Autodesk Fusion 360 part; units mm, degrees
(part 14 of 14)
sketch "Gear Tooth" plane through (0, 0, 0) normal (0, 0, 1) x (1, 0, 0)
  spline S0 degree 5 poles (44.1435, -1.3961) (44.1546, -1.396) (44.1768, -1.3957) (44.2102, -1.3951) (44.2546, -1.3938) (44.3102, -1.3914) (44.3658, -1.3882) (44.4214, -1.3842) (44.477, -1.3795) (44.5325, -1.3742) (44.5881, -1.3682) (44.6437, -1.3617) (44.6992, -1.3548) (44.7548, -1.3474) (44.8103, -1.3396) (44.8658, -1.3315) (44.9213, -1.3229) (44.9768, -1.314) (45.0323, -1.3047) (45.0878, -1.295) (45.1432, -1.285) (45.1987, -1.2746) (45.2541, -1.2639) (45.3095, -1.2528) (45.3649, -1.2415) (45.4203, -1.2298) (45.4756, -1.2179) (45.5309, -1.2056) (45.5863, -1.1931) (45.6416, -1.1803) (45.6969, -1.1672) (45.7521, -1.1538) (45.8074, -1.1401) (45.8626, -1.1262) (45.9178, -1.112) (45.973, -1.0975) (46.0282, -1.0828) (46.0833, -1.0678) (46.1384, -1.0526) (46.1935, -1.0371) (46.2486, -1.0214) (46.3037, -1.0055) (46.3587, -0.9893) (46.4137, -0.9728) (46.4687, -0.9562) (46.5237, -0.9393) (46.5786, -0.9222) (46.6336, -0.9048) (46.6885, -0.8872) (46.7433, -0.8694) (46.7982, -0.8514) (46.853, -0.8332) (46.9078, -0.8147) (46.9626, -0.796) (47.0173, -0.7771) (47.0721, -0.758) (47.1268, -0.7387) (47.1814, -0.7192) (47.2361, -0.6995) (47.2907, -0.6796) (47.3453, -0.6595) (47.3999, -0.6391) (47.4544, -0.6186) (47.5089, -0.5979) (47.5634, -0.5769) (47.6179, -0.5558) (47.6723, -0.5345) (47.7267, -0.513) (47.7811, -0.4913) (47.8354, -0.4694) (47.8898, -0.4473) (47.9332, -0.4295) (47.9658, -0.416) (47.9875, -0.407) (47.9983, -0.4025) knots 0 0 0 0 0 0 0.01428571 0.02857143 0.04285714 0.05714286 0.07142857 0.08571429 0.1 0.11428571 0.12857143 0.14285714 0.15714286 0.17142857 0.18571429 0.2 0.21428571 0.22857143 0.24285714 0.25714286 0.27142857 0.28571429 0.3 0.31428571 0.32857143 0.34285714 0.35714286 0.37142857 0.38571429 0.4 0.41428571 0.42857143 0.44285714 0.45714286 0.47142857 0.48571429 0.5 0.51428571 0.52857143 0.54285714 0.55714286 0.57142857 0.58571429 0.6 0.61428571 0.62857143 0.64285714 0.65714286 0.67142857 0.68571429 0.7 0.71428571 0.72857143 0.74285714 0.75714286 0.77142857 0.78571429 0.8 0.81428571 0.82857143 0.84285714 0.85714286 0.87142857 0.88571429 0.9 0.91428571 0.92857143 0.94285714 0.95714286 0.97142857 0.98571429 1 1 1 1 1 1
  spline S1 degree 5 poles (44.1435, 1.3961) (44.1546, 1.396) (44.1768, 1.3957) (44.2102, 1.3951) (44.2546, 1.3938) (44.3102, 1.3914) (44.3658, 1.3882) (44.4214, 1.3842) (44.477, 1.3795) (44.5325, 1.3742) (44.5881, 1.3682) (44.6437, 1.3617) (44.6992, 1.3548) (44.7548, 1.3474) (44.8103, 1.3396) (44.8658, 1.3315) (44.9213, 1.3229) (44.9768, 1.314) (45.0323, 1.3047) (45.0878, 1.295) (45.1432, 1.285) (45.1987, 1.2746) (45.2541, 1.2639) (45.3095, 1.2528) (45.3649, 1.2415) (45.4203, 1.2298) (45.4756, 1.2179) (45.5309, 1.2056) (45.5863, 1.1931) (45.6416, 1.1803) (45.6969, 1.1672) (45.7521, 1.1538) (45.8074, 1.1401) (45.8626, 1.1262) (45.9178, 1.112) (45.973, 1.0975) (46.0282, 1.0828) (46.0833, 1.0678) (46.1384, 1.0526) (46.1935, 1.0371) (46.2486, 1.0214) (46.3037, 1.0055) (46.3587, 0.9893) (46.4137, 0.9728) (46.4687, 0.9562) (46.5237, 0.9393) (46.5786, 0.9222) (46.6336, 0.9048) (46.6885, 0.8872) (46.7433, 0.8694) (46.7982, 0.8514) (46.853, 0.8332) (46.9078, 0.8147) (46.9626, 0.796) (47.0173, 0.7771) (47.0721, 0.758) (47.1268, 0.7387) (47.1814, 0.7192) (47.2361, 0.6995) (47.2907, 0.6796) (47.3453, 0.6595) (47.3999, 0.6391) (47.4544, 0.6186) (47.5089, 0.5979) (47.5634, 0.5769) (47.6179, 0.5558) (47.6723, 0.5345) (47.7267, 0.513) (47.7811, 0.4913) (47.8354, 0.4694) (47.8898, 0.4473) (47.9332, 0.4295) (47.9658, 0.416) (47.9875, 0.407) (47.9983, 0.4025) knots 0 0 0 0 0 0 0.01428571 0.02857143 0.04285714 0.05714286 0.07142857 0.08571429 0.1 0.11428571 0.12857143 0.14285714 0.15714286 0.17142857 0.18571429 0.2 0.21428571 0.22857143 0.24285714 0.25714286 0.27142857 0.28571429 0.3 0.31428571 0.32857143 0.34285714 0.35714286 0.37142857 0.38571429 0.4 0.41428571 0.42857143 0.44285714 0.45714286 0.47142857 0.48571429 0.5 0.51428571 0.52857143 0.54285714 0.55714286 0.57142857 0.58571429 0.6 0.61428571 0.62857143 0.64285714 0.65714286 0.67142857 0.68571429 0.7 0.71428571 0.72857143 0.74285714 0.75714286 0.77142857 0.78571429 0.8 0.81428571 0.82857143 0.84285714 0.85714286 0.87142857 0.88571429 0.9 0.91428571 0.92857143 0.94285714 0.95714286 0.97142857 0.98571429 1 1 1 1 1 1
  arc A0 (47.9983, -0.4025) -> (47.9983, 0.4025) centre (0, 0) ccw
  line L0 (44.1435, 1.3961) -> (44.1435, -1.3961)
  point P0 (44.4179, -1.3843)
  point P1 (44.6928, -1.3555)
  point P2 (44.968, -1.3153)
  point P3 (45.2434, -1.2659)
  point P4 (45.519, -1.2082)
  point P5 (45.7946, -1.1432)
  point P6 (46.0703, -1.0713)
  point P7 (46.346, -0.993)
  point P8 (46.6217, -0.9085)
  point P9 (46.8973, -0.8182)
  point P10 (47.1728, -0.7223)
  point P11 (47.4482, -0.6209)
  point P12 (47.7233, -0.5143)
  point P13 (44.4179, 1.3843)
  point P14 (44.6928, 1.3555)
  point P15 (44.968, 1.3153)
  point P16 (45.2434, 1.2659)
  point P17 (45.519, 1.2082)
  point P18 (45.7946, 1.1432)
  point P19 (46.0703, 1.0713)
  point P20 (46.346, 0.993)
  point P21 (46.6217, 0.9085)
  point P22 (46.8973, 0.8182)
  point P23 (47.1728, 0.7223)
  point P24 (47.4482, 0.6209)
  point P25 (47.7233, 0.5143)
extrude "Extrude2" add sketch "Gear Tooth" along normal blind 6
fillet "Fillet1" radius 0.38 2 edges at (45.829, 1.1346, 3) (45.829, -1.1346, 3)
pattern_circular "C-Pattern1" count 94 over 360 about axis through (0, 0, 0) along (0, 0, 1) of "Extrude2", "Fillet1"
sketch "Diametrial Pitch Circle" plane through (0, 0, 0) normal (0, 0, 1) x (1, 0, 0)
  circle A0 centre (0, 0) radius 47 construction
named bodies: "Spur Gear (94 teeth)"

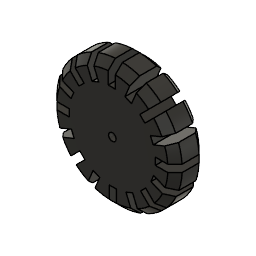
design "car project wheels"
part number: 2026-02-16-19-34-30-202
Autodesk Fusion 360 part; units mm, degrees
sketch "Sketch1" plane through (0, 0, 0) normal (0, 0, 1) x (1, 0, 0)
  circle A0 centre (0, 0) radius 2.1
  circle A1 centre (0, 0) radius 35
  dimension "d1" = 4.2
  dimension "d2" = 70
  constraint coincident A0.centre A1.centre
  measures "d1" diameter of A0
  measures "d2" diameter of A1
extrude "Extrude1" add sketch "Sketch1" along normal blind 17.5
chamfer "Chamfer1" distance 4 angle 45 2 edges at (-32.6315, -12.6565, 17.5) (-32.6315, -12.6565, 0)
sketch "Sketch2" plane through (0, 0, 0) normal (0, 0, 1) x (1, 0, 0)
sketch "Sketch3" plane through (0, 0, 0) normal (0, 0, 1) x (1, 0, 0)
sketch "Sketch5" plane through (0, 0, 0) normal (0, 0, 1) x (1, 0, 0)
  line L0 (-0.313, 36) -> (1.687, 36)
  line L1 (1.687, 36) -> (1.687, 24)
  line L2 (1.687, 24) -> (-2.313, 24)
  line L3 (-2.313, 24) -> (-2.313, 36)
  line L4 (-2.313, 36) -> (-0.313, 36)
  dimension "d17" = 2
  dimension "d18" = 12
  dimension "d19" = 4
  dimension "d20" = 12
  constraint horizontal L0
  constraint perpendicular L0 L1
  constraint perpendicular L1 L2
  constraint perpendicular L2 L3
  measures "d17" distance of L0.start L0.end
  measures "d18" distance of L0.end L1.end
  measures "d19" distance of L1.end L2.end
  measures "d20" distance of L2.end L3.end
extrude "Extrude3" cut sketch "Sketch5" along normal blind 45
pattern_circular "C-Pattern3" count 16 over 360 about axis through (0, 0, 0) along (0, 0, 1) of "Extrude3"
sketch "Sketch6" plane through (0, 0, 0) normal (0, 0, 1) x (1, 0, 0)

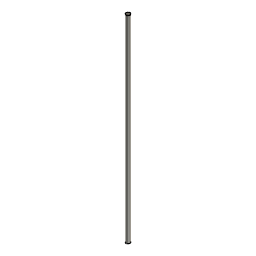
design "Axle"
part number: 2026-03-02-11-54-45-351
Autodesk Fusion 360 part; units mm, degrees
sketch "Sketch1" plane through (0, 0, 0) normal (0, 0, 1) x (1, 0, 0)
  circle A0 centre (0, 0) radius 2
  dimension "d1" = 4
  constraint coincident A0.centre origin
  measures "d1" diameter of A0
extrude "Extrude1" add sketch "Sketch1" along normal blind 190

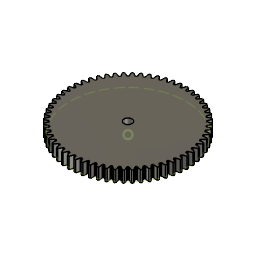
design "60 compound gear"
description: Spur Gear; Module: 1.0; Num Teeth: 60; Pressure Angle: 20.0; Backlash: 0.00 mm
part number: 2026-09-03-00-53-56-789
Autodesk Fusion 360 part; units mm, degrees
sketch "Base Circle" plane through (0, 0, 0) normal (0, 0, 1) x (1, 0, 0)
  circle A0 centre (0, 0) radius 28.843
  circle A1 centre (0, 0) radius 2.1
extrude "Extrude1" add sketch "Base Circle" along normal blind 6
sketch "Gear Tooth" plane through (0, 0, 0) normal (0, 0, 1) x (1, 0, 0)
  spline S0 degree 5 poles (28.167, -1.1579) (28.1751, -1.1579) (28.1914, -1.1578) (28.2159, -1.1575) (28.2485, -1.1567) (28.2892, -1.1551) (28.33, -1.1529) (28.3707, -1.1501) (28.4115, -1.1467) (28.4523, -1.1427) (28.493, -1.1383) (28.5338, -1.1335) (28.5746, -1.1284) (28.6154, -1.1228) (28.6561, -1.117) (28.6969, -1.1109) (28.7376, -1.1045) (28.7783, -1.0977) (28.8191, -1.0907) (28.8598, -1.0834) (28.9005, -1.0758) (28.9412, -1.0679) (28.9819, -1.0597) (29.0226, -1.0513) (29.0633, -1.0427) (29.104, -1.0338) (29.1446, -1.0247) (29.1853, -1.0153) (29.2259, -1.0057) (29.2665, -0.9959) (29.3071, -0.9858) (29.3477, -0.9755) (29.3883, -0.965) (29.4289, -0.9543) (29.4694, -0.9434) (29.5099, -0.9323) (29.5505, -0.921) (29.591, -0.9094) (29.6315, -0.8977) (29.672, -0.8858) (29.7124, -0.8737) (29.7529, -0.8614) (29.7933, -0.8488) (29.8337, -0.8361) (29.8741, -0.8233) (29.9145, -0.8102) (29.9549, -0.7969) (29.9952, -0.7835) (30.0355, -0.7699) (30.0759, -0.7561) (30.1161, -0.7421) (30.1564, -0.728) (30.1967, -0.7137) (30.2369, -0.6992) (30.2771, -0.6845) (30.3173, -0.6697) (30.3575, -0.6547) (30.3977, -0.6396) (30.4378, -0.6242) (30.4779, -0.6087) (30.518, -0.5931) (30.5581, -0.5773) (30.5982, -0.5613) (30.6382, -0.5451) (30.6782, -0.5288) (30.7182, -0.5124) (30.7582, -0.4958) (30.7981, -0.479) (30.838, -0.4621) (30.8779, -0.445) (30.9178, -0.4278) (30.9497, -0.4139) (30.9736, -0.4034) (30.9895, -0.3963) (30.9975, -0.3928) knots 0 0 0 0 0 0 0.01428571 0.02857143 0.04285714 0.05714286 0.07142857 0.08571429 0.1 0.11428571 0.12857143 0.14285714 0.15714286 0.17142857 0.18571429 0.2 0.21428571 0.22857143 0.24285714 0.25714286 0.27142857 0.28571429 0.3 0.31428571 0.32857143 0.34285714 0.35714286 0.37142857 0.38571429 0.4 0.41428571 0.42857143 0.44285714 0.45714286 0.47142857 0.48571429 0.5 0.51428571 0.52857143 0.54285714 0.55714286 0.57142857 0.58571429 0.6 0.61428571 0.62857143 0.64285714 0.65714286 0.67142857 0.68571429 0.7 0.71428571 0.72857143 0.74285714 0.75714286 0.77142857 0.78571429 0.8 0.81428571 0.82857143 0.84285714 0.85714286 0.87142857 0.88571429 0.9 0.91428571 0.92857143 0.94285714 0.95714286 0.97142857 0.98571429 1 1 1 1 1 1
  spline S1 degree 5 poles (28.167, 1.1579) (28.1751, 1.1579) (28.1914, 1.1578) (28.2159, 1.1575) (28.2485, 1.1567) (28.2892, 1.1551) (28.33, 1.1529) (28.3707, 1.1501) (28.4115, 1.1467) (28.4523, 1.1427) (28.493, 1.1383) (28.5338, 1.1335) (28.5746, 1.1284) (28.6154, 1.1228) (28.6561, 1.117) (28.6969, 1.1109) (28.7376, 1.1045) (28.7783, 1.0977) (28.8191, 1.0907) (28.8598, 1.0834) (28.9005, 1.0758) (28.9412, 1.0679) (28.9819, 1.0597) (29.0226, 1.0513) (29.0633, 1.0427) (29.104, 1.0338) (29.1446, 1.0247) (29.1853, 1.0153) (29.2259, 1.0057) (29.2665, 0.9959) (29.3071, 0.9858) (29.3477, 0.9755) (29.3883, 0.965) (29.4289, 0.9543) (29.4694, 0.9434) (29.5099, 0.9323) (29.5505, 0.921) (29.591, 0.9094) (29.6315, 0.8977) (29.672, 0.8858) (29.7124, 0.8737) (29.7529, 0.8614) (29.7933, 0.8488) (29.8337, 0.8361) (29.8741, 0.8233) (29.9145, 0.8102) (29.9549, 0.7969) (29.9952, 0.7835) (30.0355, 0.7699) (30.0759, 0.7561) (30.1161, 0.7421) (30.1564, 0.728) (30.1967, 0.7137) (30.2369, 0.6992) (30.2771, 0.6845) (30.3173, 0.6697) (30.3575, 0.6547) (30.3977, 0.6396) (30.4378, 0.6242) (30.4779, 0.6087) (30.518, 0.5931) (30.5581, 0.5773) (30.5982, 0.5613) (30.6382, 0.5451) (30.6782, 0.5288) (30.7182, 0.5124) (30.7582, 0.4958) (30.7981, 0.479) (30.838, 0.4621) (30.8779, 0.445) (30.9178, 0.4278) (30.9497, 0.4139) (30.9736, 0.4034) (30.9895, 0.3963) (30.9975, 0.3928) knots 0 0 0 0 0 0 0.01428571 0.02857143 0.04285714 0.05714286 0.07142857 0.08571429 0.1 0.11428571 0.12857143 0.14285714 0.15714286 0.17142857 0.18571429 0.2 0.21428571 0.22857143 0.24285714 0.25714286 0.27142857 0.28571429 0.3 0.31428571 0.32857143 0.34285714 0.35714286 0.37142857 0.38571429 0.4 0.41428571 0.42857143 0.44285714 0.45714286 0.47142857 0.48571429 0.5 0.51428571 0.52857143 0.54285714 0.55714286 0.57142857 0.58571429 0.6 0.61428571 0.62857143 0.64285714 0.65714286 0.67142857 0.68571429 0.7 0.71428571 0.72857143 0.74285714 0.75714286 0.77142857 0.78571429 0.8 0.81428571 0.82857143 0.84285714 0.85714286 0.87142857 0.88571429 0.9 0.91428571 0.92857143 0.94285714 0.95714286 0.97142857 0.98571429 1 1 1 1 1 1
  arc A0 (30.9975, -0.3928) -> (30.9975, 0.3928) centre (0, 0) ccw
  line L0 (28.167, 1.1579) -> (28.167, -1.1579)
  point P0 (28.3681, -1.1501)
  point P1 (28.5698, -1.1289)
  point P2 (28.7718, -1.0988)
  point P3 (28.974, -1.0613)
  point P4 (29.1763, -1.0173)
  point P5 (29.3788, -0.9675)
  point P6 (29.5813, -0.9122)
  point P7 (29.7839, -0.8517)
  point P8 (29.9864, -0.7864)
  point P9 (30.1889, -0.7164)
  point P10 (30.3912, -0.6419)
  point P11 (30.5935, -0.5631)
  point P12 (30.7956, -0.48)
  point P13 (28.3681, 1.1501)
  point P14 (28.5698, 1.1289)
  point P15 (28.7718, 1.0988)
  point P16 (28.974, 1.0613)
  point P17 (29.1763, 1.0173)
  point P18 (29.3788, 0.9675)
  point P19 (29.5813, 0.9122)
  point P20 (29.7839, 0.8517)
  point P21 (29.9864, 0.7864)
  point P22 (30.1889, 0.7164)
  point P23 (30.3912, 0.6419)
  point P24 (30.5935, 0.5631)
  point P25 (30.7956, 0.48)
extrude "Extrude2" add sketch "Gear Tooth" along normal blind 6
fillet "Fillet1" radius 0.38 2 edges at (28.8224, 1.09, 3) (28.8224, -1.09, 3)
pattern_circular "C-Pattern1" count 60 over 360 about axis through (0, 0, 0) along (0, 0, 1) of "Extrude2", "Fillet1"
sketch "Diametrial Pitch Circle" plane through (0, 0, 0) normal (0, 0, 1) x (1, 0, 0)
  circle A0 centre (0, 0) radius 30 construction
named bodies: "Spur Gear (60 teeth)"

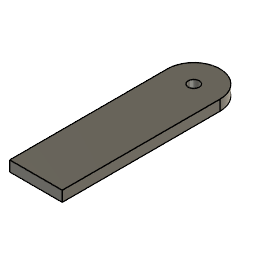
design "prong"
part number: 2026-03-17-23-28-56-829
Autodesk Fusion 360 part; units mm, degrees
sketch "Sketch1" plane through (0, 0, 0) normal (0, 0, 1) x (1, 0, 0)
  line L0 (-10, 0) -> (-10, -60)
  line L1 (-10, -60) -> (10, -60)
  line L2 (10, -60) -> (10, 0)
  arc A0 (10, 0) -> (-10, 0) centre (0, 0) ccw
  dimension "d1" = 20
  dimension "d2" = 60
  constraint coincident A0.centre origin
  constraint vertical L0
  constraint perpendicular L0 L1
  constraint tangent L2 A0
  constraint perpendicular L1 L2
  measures "d1" diameter of A0
  measures "d2" distance of L0.start L0.end
extrude "Extrude1" add sketch "Sketch1" along normal blind 4
sketch "Sketch2" plane through (0, 0, 4) normal (0, 0, 1) x (-1, 0, 0)
  arc A0 (-10, 0) -> (10, 0) centre (0, 0) ccw
  line L0 (10, 0) -> (10, 60)
  line L1 (10, 60) -> (-10, 60)
  line L2 (-10, 60) -> (-10, 0)
  circle A1 centre (0, 0) radius 2.1
  dimension "d5" = 4.2
  constraint coincident A0.centre A1.centre
  measures "d5" diameter of A1
extrude "Extrude2" cut sketch "Sketch2" against normal blind 4 contours A1

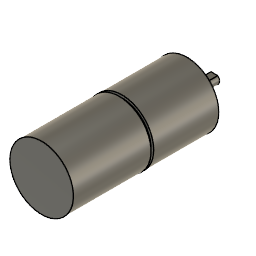
design "DC motor - gearbox"
part number: 2026-02-09-11-49-54-092
Autodesk Fusion 360 part; units mm, degrees
sketch "Sketch1" plane through (0, 0, 0) normal (0, 1, 0) x (1, 0, 0)
  circle A0 centre (0, 0) radius 12.2
  dimension "d1" = 24.4
  constraint coincident A0.centre origin
  measures "d1" diameter of A0
extrude "Extrude1" add sketch "Sketch1" along normal blind 30.8
sketch "Sketch2" plane through (0, 30.8, 0) normal (0, 1, 0) x (-1, 0, 0)
  circle A0 centre (0, 0) radius 12.2
  circle A1 centre (0, 0) radius 12.5
  dimension "d4" = 25
  constraint concentric A0 A1
  measures "d4" diameter of A1
chamfer "Chamfer1" distance 1 angle 45 1 edges at (-11.3744, 30.8, 4.4117)
extrude "Extrude2" add sketch "Sketch2" along normal blind 25 contours A0
sketch "Sketch3" plane through (0, 55.8, 0) normal (0, 1, 0) x (-1, 0, 0)
  circle A0 centre (0, 0) radius 12.2
  circle A1 centre (0, 0) radius 3.5
  dimension "d8" = 7
  constraint concentric A0 A1
  measures "d8" diameter of A1
extrude "Extrude3" add sketch "Sketch3" along normal blind 2.5 contours A1
sketch "Sketch4" plane through (0, 58.3, 0) normal (0, 1, 0) x (-1, 0, 0)
  circle A0 centre (0, 0) radius 3.5
  circle A1 centre (0, 0) radius 2
  dimension "d11" = 4
  constraint concentric A0 A1
  measures "d11" diameter of A1
extrude "Extrude4" add sketch "Sketch4" along normal blind 8 contours A1
sketch "Sketch5" plane through (0, 66.3, 0) normal (0, 1, 0) x (-1, 0, 0)
  circle A0 centre (0, 0) radius 2
  line L0 (-1.3229, 1.5) -> (1.3229, 1.5)
  constraint coincident A0 L0.start
  constraint coincident A0 L0.end
extrude "Extrude5" cut sketch "Sketch5" against normal blind 8 contours A0 L0 picked at (-0.3643, 1.5583)
